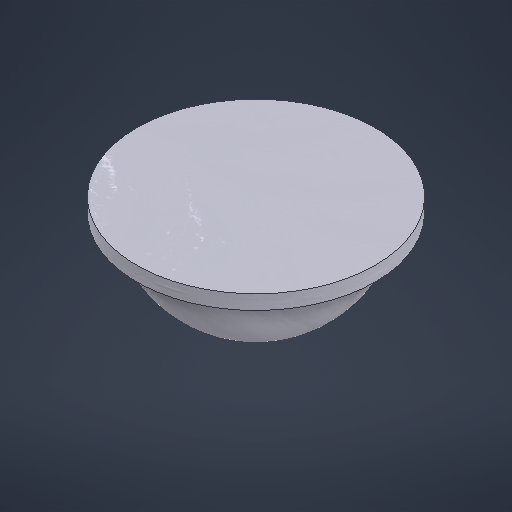
# Autodesk Inventor part: OGCasterWheel
Saved by Autodesk Inventor 2027 (Build 310192060, 192F)
## iProperties
Created: 2026-07-12
Part Number: OGCasterWheel
Material: Stainless Steel AISI 440C, Welded
Document SubType Name: Modeling
Designer: machnach0
Density: 7.8 g/cm^3
Appearance: Weld - Stainless Steel
Author: machnach0
Autodesk Inventor part; units mm, degrees
ref_plane "YZ Plane" through (0, 0, 0) normal (1, 0, 0) x (0, 1, 0)
ref_plane "XZ Plane" through (0, 0, 0) normal (0, 1, 0) x (-1, 0, 0)
ref_plane "XY Plane" through (0, 0, 0) normal (0, 0, 1) x (1, 0, 0)
sketch "Sketch1" plane through (0, 0, 0) normal (0, 0, 1) x (1, 0, 0)
  line L0 (0, 0) -> (22.0374, 0)
  arc A0 (0, -19.05) -> (18.8624, -2.667) centre (0, 0) ccw
  line L1 (18.8624, -2.667) -> (22.0374, -2.667)
  line L2 (22.0374, -2.667) -> (22.0374, 0)
  line L3 (0, 0) -> (0, -19.05)
  dimension "d0" = 3.175
  dimension "d1" = 19.05
  dimension "d2" = 2.667
  constraints: 8 end point, 2 horizontal, 2 point on circle, 1 centre point, 1 coincident, 1 parallel, 1 perpendicular
  measures "d0" distance of L1.start L1.end
  measures "d1" distance of L3.start L3.end
  measures "d2" distance of L1.end L0.end
revolve "Revolution1" add sketch "Sketch1" angle 360 about axis through (0, 0, 0) along (0, -1, 0)
body "Solid1"
